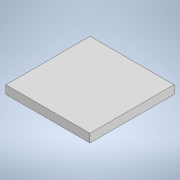
# Autodesk Inventor part: Red Alliance Marker
Saved by Autodesk Inventor 2020 (Build 240168000, 168)
## iProperties
Created: 2020-01-13
Part Number: Red Alliance Marker
Material: Generic
Document SubType Name: Modeling
Designer: maple
Density: 1 g/cm^3
Appearance: Default
Author: maple
Autodesk Inventor part; units mm, degrees
ref_plane "YZ Plane" through (0, 0, 0) normal (1, 0, 0) x (0, 1, 0)
ref_plane "XZ Plane" through (0, 0, 0) normal (0, 1, 0) x (-1, 0, 0)
ref_plane "XY Plane" through (0, 0, 0) normal (0, 0, 1) x (1, 0, 0)
sketch "Sketch1" plane through (0, 0, 0) normal (0, 1, 0) x (-1, 0, 0)
  line L0 (0, 0) -> (-63.5, 0)
  line L1 (-63.5, 0) -> (-63.5, -63.5)
  line L2 (-63.5, -63.5) -> (0, -63.5)
  line L3 (0, -63.5) -> (0, 0)
  dimension "d0" = 63.5
  dimension "d1" = 63.5
  constraints: 8 end point, 2 parallel, 1 horizontal, 1 perpendicular
  measures "d0" distance of L2.end L1.end
  measures "d1" distance of L1.end L0.end
extrude "Extrusion1" add sketch "Sketch1" along normal blind 6.35
sketch "Sketch4" plane through (0, 0, 0) normal (0, -1, 0) x (1, 0, 0)
  line L0 (1.5686, -1.4924) -> (9.3639, -1.4924) construction
  line L1 (9.3639, -1.4924) -> (9.3639, -4.5404) construction
  line L2 (9.3639, -4.5404) -> (1.5686, -4.5404) construction
  line L3 (1.5686, -4.5404) -> (1.5686, -1.4924) construction
  line L4 (4.2362, -4.5404) -> (3.7101, -4.5404)
  line L5 (3.7101, -4.5404) -> (2.7468, -3.3276)
  line L6 (2.7468, -3.3276) -> (2.2824, -3.3276)
  line L7 (2.2824, -3.3276) -> (2.2824, -4.5404)
  line L8 (2.2824, -4.5404) -> (1.8773, -4.5404)
  line L9 (1.8773, -4.5404) -> (1.8773, -1.4924)
  line L10 (1.8773, -1.4924) -> (2.6628, -1.4924)
  spline S0 degree 2 poles (2.6628, -1.4924) (2.9246, -1.4924) (3.2778, -1.5492) (3.4384, -1.6529) knots 0 0 0 1 2 2 2
  spline S1 degree 2 poles (3.4384, -1.6529) (3.5989, -1.7567) (3.7842, -2.0803) (3.7842, -2.3198) knots 0 0 0 1 2 2 2
  spline S2 degree 2 poles (3.7842, -2.3198) (3.7842, -2.6533) (3.4433, -3.1053) (3.1518, -3.214) knots 0 0 0 1 2 2 2
  line L11 (3.1518, -3.214) -> (4.2362, -4.5404)
  spline S3 degree 2 poles (3.3618, -2.352) (3.3618, -2.2186) (3.2679, -2.0136) (3.1691, -1.9469) knots 0 0 0 1 2 2 2
  spline S4 degree 2 poles (3.1691, -1.9469) (3.0827, -1.8901) (2.853, -1.8431) (2.685, -1.8431) knots 0 0 0 1 2 2 2
  line L12 (2.685, -1.8431) -> (2.2824, -1.8431)
  line L13 (2.2824, -1.8431) -> (2.2824, -2.9892)
  line L14 (2.2824, -2.9892) -> (2.6381, -2.9892)
  spline S5 degree 2 poles (2.6381, -2.9892) (2.8134, -2.9892) (3.0926, -2.9275) (3.1889, -2.8311) knots 0 0 0 1 2 2 2
  spline S6 degree 2 poles (3.1889, -2.8311) (3.2778, -2.7472) (3.3618, -2.51) (3.3618, -2.352) knots 0 0 0 1 2 2 2
  line L15 (4.4782, -4.5404) -> (4.4782, -1.4924)
  line L16 (4.4782, -1.4924) -> (6.3851, -1.4924)
  line L17 (6.3851, -1.4924) -> (6.3851, -1.853)
  line L18 (6.3851, -1.853) -> (4.8833, -1.853)
  line L19 (4.8833, -1.853) -> (4.8833, -2.6879)
  line L20 (4.8833, -2.6879) -> (6.2838, -2.6879)
  line L21 (6.2838, -2.6879) -> (6.2838, -3.0485)
  line L22 (6.2838, -3.0485) -> (4.8833, -3.0485)
  line L23 (4.8833, -3.0485) -> (4.8833, -4.1798)
  line L24 (4.8833, -4.1798) -> (6.3851, -4.1798)
  line L25 (6.3851, -4.1798) -> (6.3851, -4.5404)
  line L26 (6.3851, -4.5404) -> (4.4782, -4.5404)
  spline S7 degree 2 poles (9.233, -3.0189) (9.233, -3.4363) (8.8946, -4.1081) (8.6106, -4.2959) knots 0 0 0 1 2 2 2
  spline S8 degree 2 poles (8.6106, -4.2959) (8.3784, -4.4416) (7.9017, -4.5404) (7.5312, -4.5404) knots 0 0 0 1 2 2 2
  line L27 (7.5312, -4.5404) -> (6.8297, -4.5404)
  line L28 (6.8297, -4.5404) -> (6.8297, -1.4924)
  line L29 (6.8297, -1.4924) -> (7.5238, -1.4924)
  spline S9 degree 2 poles (7.5238, -1.4924) (7.9535, -1.4924) (8.4426, -1.6208) (8.6155, -1.7345) knots 0 0 0 1 2 2 2
  spline S10 degree 2 poles (8.6155, -1.7345) (8.9094, -1.9296) (9.233, -2.5743) (9.233, -3.0189) knots 0 0 0 1 2 2 2
  spline S11 degree 2 poles (8.8106, -3.0139) (8.8106, -2.6632) (8.5785, -2.1667) (8.3488, -2.0259) knots 0 0 0 1 2 2 2
  spline S12 degree 2 poles (8.3488, -2.0259) (8.1857, -1.9296) (7.8177, -1.8431) (7.5435, -1.8431) knots 0 0 0 1 2 2 2
  line L30 (7.5435, -1.8431) -> (7.2348, -1.8431)
  line L31 (7.2348, -1.8431) -> (7.2348, -4.1897)
  line L32 (7.2348, -4.1897) -> (7.5435, -4.1897)
  spline S13 degree 2 poles (7.5435, -4.1897) (7.8128, -4.1897) (8.2203, -4.1032) (8.3858, -3.9871) knots 0 0 0 1 2 2 2
  spline S14 degree 2 poles (8.3858, -3.9871) (8.5982, -3.8438) (8.8106, -3.3696) (8.8106, -3.0139) knots 0 0 0 1 2 2 2
  point P0 (0, 0)
  constraints: 2 other
emboss "Emboss2" sketch "Sketch4" operation add depth 0.508 direction (0, 1, 0)
body "Solid1"
